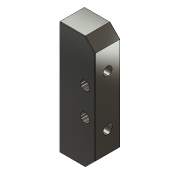
# Autodesk Inventor part: BC-10008
Saved by Autodesk Inventor 2016 (Build 200138000, 138)
## iProperties
Created: 2015-11-25
Part Number: BC-10008
Material: Aço Carbono AISI 1006
Document SubType Name: Modeling
Designer: reinaldo.basilio!
Density: 7.87 g/cm^3
Appearance: Silver
Mass: 5716.2 g
Surface Area: 701.193 cm^2
Volume: 726.328 cm^3
Project: DIPOLO BC-3T- SIRIUS
Description: Peça frontal inferior para fechar circuito  magnético.
Author: reinaldo.basilio
Title: DIPOLO BC-3T- SIRIUS
Subject: BC-10008
Autodesk Inventor part; units mm, degrees
ref_plane "YZ Plane" through (0, 0, 0) normal (1, 0, 0) x (0, 1, 0)
ref_plane "XZ Plane" through (0, 0, 0) normal (0, 1, 0) x (-1, 0, 0)
ref_plane "XY Plane" through (0, 0, 0) normal (0, 0, 1) x (1, 0, 0)
sketch "Sketch1" plane through (0, 0, 0) normal (0, 1, 0) x (-1, 0, 0)
  line L0 (35, 112.5) -> (-35, 112.5)
  line L1 (-35, 112.5) -> (-35, -112.5)
  line L2 (-35, -112.5) -> (35, -112.5)
  line L3 (35, -112.5) -> (35, 112.5)
  point P0 (0, 0)
  point P1 (35, 0)
  point P2 (0, -112.5)
  dimension "d0" = 225
  dimension "d1" = 70
  constraints: 8 end point, 2 midpoint, 2 parallel, 1 horizontal, 1 horizontal alignment, 1 perpendicular, 1 vertical alignment
  measures "d0" distance of L2.end L0.start
  measures "d1" distance of L0.start L0.end
extrude "Extrusion1" add sketch "Sketch1" along normal blind 50
sketch "Sketch2" plane through (35, 0, 112.5) normal (1, 0, 0) x (0, 0, -1)
  circle A0 centre (62.5, 25) radius 5
  circle A1 centre (162.5, 25) radius 5
  line L0 (225, 0) -> (225, 50) projected
  point P0 (0, 50)
  point P1 (112.5, 0)
  point P2 (225, 25)
  dimension "d5" = 50
  dimension "d6" = 50
  dimension "d8" = 225
  dimension "d33" = 10
  constraints: 2 centre point, 2 horizontal alignment, 1 equal radius, 1 midpoint
  measures "d5" horizontal distance of A0.centre point (112.5, 0)
  measures "d6" horizontal distance of A1.centre point (112.5, 0)
  measures "d8" distance of point (0, 50) L0.end
  measures "d33" diameter of A0
hole "Hole1" at (35, 25, 50) at (35, 25, -50) direction (-1, 0, 0) diameter 10.5 end through all counterbore diameter 18 counterbore depth 35 clearance for "Socket Head Cap Screw DIN EN ISO 4762" size "M10" standard "DIN"
sketch "Sketch3" plane through (0, 0, 0) normal (0, -1, 0) x (1, 0, 0)
  line L0 (35, 112.5) -> (35, -112.5) projected
  circle A0 centre (15, 27.5) radius 5
  circle A1 centre (15, -27.5) radius 5
  point P0 (0, 0)
  dimension "d17" = 55
  dimension "d18" = 20
  dimension "d21" = 27.5
  dimension "d32" = 10
  constraints: 2 centre point, 1 equal radius, 1 vertical alignment
  measures "d17" distance of A0.centre A1.centre
  measures "d18" distance from line of L0 A1.centre
  measures "d21" vertical distance of point (0, 0) A0.centre
  measures "d32" diameter of A0
hole "Hole2" at (15, 0, 27.5) at (15, 0, -27.5) direction (0, 1, 0) diameter 10.5 end through all counterbore diameter 18 counterbore depth 15 clearance for "Socket Head Cap Screw DIN EN ISO 4762" size "M10" standard "DIN"
chamfer "Chamfer1" distance 20 angle 45 2 edges at (35, 25, 112.5) (35, 25, -112.5)
sketch "Sketch4" plane through (0, 50, 0) normal (0, 1, 0) x (1, 0, 0)
  line L0 (-35, 112.5) -> (-35, -112.5) projected
  circle A0 centre (-27.5, -103.5) radius 4
  circle A1 centre (-27.5, -76.5) radius 4
  circle A2 centre (-14, -90) radius 4
  line L1 (0, 0) -> (7.2062, 0) construction
  circle A3 centre (-27.5, 103.5) radius 4
  circle A4 centre (-27.5, 76.5) radius 4
  circle A5 centre (-14, 90) radius 4
  dimension "d36" = 13.5
  dimension "d37" = 27
  dimension "d38" = 8
  dimension "d39" = 7.5
  dimension "d40" = 8
  dimension "d41" = 90
  dimension "d42" = 13.5
  constraints: 6 centre point, 3 symmetric about line, 2 end point, 2 equal radius, 1 horizontal, 1 vertical alignment, 3 other
  measures "d36" horizontal distance of A1.centre A2.centre
  measures "d37" distance of A1.centre A0.centre
  measures "d38" diameter of A0
  measures "d39" distance from line of L0 A0.centre
  measures "d40" diameter of A1
  measures "d41" distance from line of L1 A2.centre
  measures "d42" horizontal distance of A2.centre A0.centre
hole "Hole3" at (-27.5, 50, 103.5) at (-14, 50, 90) at (-27.5, 50, 76.5) at (-27.5, 50, -76.5) at (-14, 50, -90) at (-27.5, 50, -103.5) direction (0, -1, 0) diameter 6.647 depth 15 tip angle 118 thread size "M8x1.25" class "6H" standard "ISO Metric profile"
chamfer "Chamfer2" distance 1 angle 45 10 edges at (-10, 50, 112.5) (25, 50, 102.5) (35, 50, 0) (25, 50, -102.5) (-10, 50, -112.5) (-10, 0, 112.5) (25, 0, 102.5) (35, 0, 0) (25, 0, -102.5) (-10, 0, -112.5)
equation "\"d6\" = d5"
equation "\"d21\" = 0.5 * d17"
body "Solid1"
